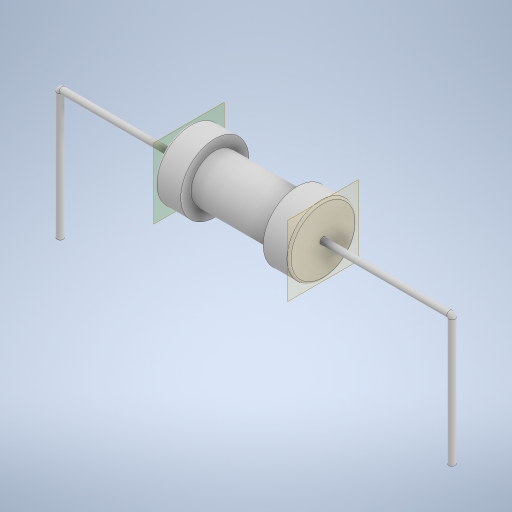
# Autodesk Inventor part: A44
Saved by Autodesk Inventor 2024 (Build 280153000, 153)
## iProperties
Created: 2023-12-15
Part Number: A44
Material: Generic
Document SubType Name: Sheet Metal
Designer: user
Density: 1 g/cm^3
Sheet Metal Rule: Default
Appearance: Default
Author: user
Autodesk Inventor part; units mm, degrees
ref_plane "YZ Plane" through (0, 0, 0) normal (1, 0, 0) x (0, 1, 0)
ref_plane "XZ Plane" through (0, 0, 0) normal (0, 1, 0) x (-1, 0, 0)
ref_plane "XY Plane" through (0, 0, 0) normal (0, 0, 1) x (1, 0, 0)
sketch "Sketch1" plane through (0, 0, 0) normal (0, 0, 1) x (1, 0, 0)
  line L0 (0, 0) -> (-13, 0)
  line L1 (-13, 0) -> (-13, 3.1)
  line L2 (-12.8, 3.3) -> (-10.5, 3.3)
  line L3 (-10.5, 3.3) -> (-10.5, 2.3)
  line L4 (-10.5, 2.3) -> (-2.5, 2.3)
  line L5 (-2.5, 2.3) -> (-2.5, 3.3)
  line L6 (-2.5, 3.3) -> (-0.2, 3.3)
  line L7 (0, 3.1) -> (0, 0)
  arc A0 (-12.8, 3.3) -> (-13, 3.1) centre (-12.8, 3.1) ccw
  arc A1 (0, 3.1) -> (-0.2, 3.3) centre (-0.2, 3.1) ccw
  line L8 (-10.5, 2.3) -> (-10.5, 0)
  line L9 (-2.5, 2.3) -> (-2.5, 0)
  point P0 (-13, 3.3)
  point P1 (0, 3.3)
  dimension "d0" = 13
  dimension "d1" = 3.3
  dimension "d2" = 2.5
  dimension "d3" = 1
  dimension "d5" = 8
  dimension "d6" = 1
  dimension "d7" = 2.5
  dimension "d8" = 0.2
  constraints: 20 end point, 7 perpendicular, 6 point on line, 4 point on circle, 4 tangent, 2 centre point, 2 horizontal, 1 equal radius
  measures "d0" distance of L0.start L0.end
  measures "d1" distance of L0.end point (-13, 3.3)
  measures "d2" distance of point (-13, 3.3) L2.end
  measures "d3" distance of L2.end L3.end
  measures "d5" distance of L3.end L4.end
  measures "d6" distance of L4.end L5.end
  measures "d7" distance of L5.end point (0, 3.3)
  measures "d8" radius of A0
revolve "Revolution1" add sketch "Sketch1" angle 360 about axis through (0, 0, 0) along (-1, 0, 0)
ref_plane "Work Plane1" through (0, 0, 0) normal (1, 0, 0) x (0, 0, -1)
sketch "Sketch2" plane through (0, 0, 0) normal (1, 0, 0) x (0, 0, -1)
  circle A0 centre (0, 0) radius 0.3
  dimension "d11" = 0.6
  constraints: 1 centre point, 1 coincident
  measures "d11" diameter of A0
sketch "Sketch3" plane through (0, 0, 0) normal (0, 0, 1) x (1, 0, 0)
  line L0 (0, 0) -> (12.3, 0)
  line L1 (12.5, -0.2) -> (12.5, -12.5)
  arc A0 (12.5, -0.2) -> (12.3, 0) centre (12.3, -0.2) ccw
  point P0 (12.5, 0)
  dimension "d12" = 12.5
  dimension "d13" = 12.5
  dimension "d14" = 0.2
  constraints: 4 end point, 2 point on circle, 2 point on line, 2 tangent, 1 centre point, 1 horizontal, 1 perpendicular
  measures "d12" distance of L0.start point (12.5, 0)
  measures "d13" distance of point (12.5, 0) L1.end
  measures "d14" radius of A0
sweep "Sweep1" add profiles "Sketch2" path "Sketch3"
ref_plane "Work Plane2" through (-13, 0, 0) normal (-1, 0, 0) x (0, 0, 1)
sketch "Sketch4" plane through (-13, 0, 0) normal (-1, 0, 0) x (0, 0, 1)
  circle A0 centre (0, 0) radius 0.3 projected
  circle A1 centre (0, 0) radius 0.3
  point P0 (0, 0)
  dimension "d18" = 0.6
  constraints: 1 centre point, 1 coincident
  measures "d18" diameter of A1
sketch "Sketch5" plane through (0, 0, 0) normal (0, 0, 1) x (1, 0, 0)
  line L0 (-13, 3.1) -> (-13, -3.1) projected
  line L1 (-13, 0) -> (-25.3, 0)
  line L2 (-25.5, -0.2) -> (-25.5, -12.5)
  arc A0 (-25.3, 0) -> (-25.5, -0.2) centre (-25.3, -0.2) ccw
  point P0 (0, 0)
  point P1 (-25.5, 0)
  dimension "d19" = 12.5
  dimension "d20" = 12.5
  dimension "d21" = 0.2
  constraints: 4 end point, 2 point on circle, 2 point on line, 2 tangent, 1 centre point, 1 horizontal, 1 midpoint, 1 perpendicular
  measures "d19" distance of L1.start point (-25.5, 0)
  measures "d20" distance of point (-25.5, 0) L2.end
  measures "d21" radius of A0
sweep "Sweep2" add profiles "Sketch4" path "Sketch5" path curves L1 A0 L2
equation "\"BendRadius\" = Thickness"
equation "\"BendReliefWidth\" = Thickness"
equation "\"BendReliefDepth\" = 0.5 * Thickness"
equation "\"CornerReliefSize\" = 4 * Thickness"
equation "\"MinimumRemnant\" = 2 * Thickness"
equation "\"TransitionRadius\" = BendRadius"
equation "\"JacobiRadiusSize\" = BendRadius"
equation "\"GapSize\" = Thickness"
equation "\"Thickness\" = 3.048"
body "Solid1"
